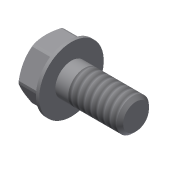
# Autodesk Inventor part: Bolt2b
Saved by Autodesk Inventor 2022.5 (Build 265521000, 521)
## iProperties
Created: 2010-08-06
Part Number: Bolt2b
Document SubType Name: Modeling
Designer: nguyenducthang
Density: 1 g/cm^3
Mass: 0.187354 g
Surface Area: 3.4646 cm^2
Volume: 0.187354 cm^3
Material: Generic
Appearance: Default
Author: nguyenducthang
Autodesk Inventor part; units mm, degrees
ref_plane "YZ Plane" through (0, 0, 0) normal (1, 0, 0) x (0, 1, 0)
ref_plane "XZ Plane" through (0, 0, 0) normal (0, 1, 0) x (-1, 0, 0)
ref_plane "XY Plane" through (0, 0, 0) normal (0, 0, 1) x (1, 0, 0)
sketch "Sketch15" plane through (0, 0, 0) normal (0, 0, 1) x (1, 0, 0)
  line L0 (0, 0) -> (0, 1.4)
  line L1 (0.2309, 1.8) -> (1.5, 1.8)
  line L2 (1.5, 1.8) -> (1.5, 2)
  line L3 (1.5, 2) -> (1.7, 2)
  line L4 (1.7, 2) -> (1.7, 1)
  line L5 (1.7, 1) -> (5.7, 1)
  line L6 (5.7, 0) -> (0, 0)
  line L7 (0.2309, 1.8) -> (0, 1.4)
  line L8 (5.7, 1) -> (5.7, 0)
  point P0 (6.0083, 0)
  dimension "d78" = 0.2
  dimension "d84" = 1
  dimension "d86" = 0.4
  dimension "d87" = 1.8
  dimension "d89" = 1.5
  dimension "d90" = 2
  dimension "d111" = 4
  constraints: 18 end point, 5 parallel, 1 perpendicular, 1 vertical, 1 other
  measures "d78" distance of L2.end L3.end
  measures "d84" distance between parallel lines of L5 L6
  measures "d86" distance from line of L0.end L1
  measures "d87" distance between parallel lines of L1 L6
  measures "d89" distance between parallel lines of L2 L0
  measures "d90" distance between parallel lines of L3 L6
  measures "d111" distance of L4.end L5.end
revolve "Revolution1" add sketch "Sketch15" angle 360 about axis through (5.7, 0, 0) along (-1, 0, 0)
chamfer "Chamfer4" distance 0.2 angle 45 1 edges at (5.7, -1, 0)
sketch "Sketch16" plane through (0, 0, 0) normal (-1, 0, 0) x (0, 0, 1)
  circle A0 centre (0, 0) radius 1.4 projected
  line L0 (0.9238, 1.6) -> (1.8475, 0)
  line L1 (1.8475, 0) -> (0.9238, -1.6)
  line L2 (0.9238, -1.6) -> (-0.9238, -1.6)
  line L3 (-0.9238, -1.6) -> (-1.8475, 0)
  line L4 (-1.8475, 0) -> (-0.9238, 1.6)
  line L5 (-0.9238, 1.6) -> (0.9238, 1.6)
  circle A1 centre (0, 0) radius 2.6573
  dimension "d104" = 3.2
  constraints: 12 end point, 2 coincident, 1 centre point, 13 other
  measures "d104" distance between parallel lines of L5 L2
extrude "Extrusion15" cut sketch "Sketch16" against normal up to surface (1.5 mm away) contours A1
thread "Thread3" size "M2x0.4" class "6g" standard "ANSI Metric M Profile" length 3
body "Solid1"
